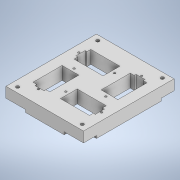
# Autodesk Inventor part: Fuehrungsgrundplatte_V2
Saved by Autodesk Inventor 2022 (Build 260153000, 153)
## iProperties
Created: 2022-04-21
Part Number: Fuehrungsgrundplatte_V2
Material: Generisch
Document SubType Name: Modeling
Designer: 123St
Density: 1 g/cm^3
Appearance: Vorgabe
Author: 123St
Autodesk Inventor part; units mm, degrees
ref_plane "YZ Plane" through (0, 0, 0) normal (1, 0, 0) x (0, 1, 0)
ref_plane "XZ Plane" through (0, 0, 0) normal (0, 1, 0) x (-1, 0, 0)
ref_plane "XY Plane" through (0, 0, 0) normal (0, 0, 1) x (1, 0, 0)
sketch "Skizze1" plane through (0, 0, 0) normal (0, 1, 0) x (-1, 0, 0)
  line L0 (30, -35) -> (-30, -35)
  line L1 (-30, -35) -> (-30, 35)
  line L2 (-30, 35) -> (30, 35)
  line L3 (30, 35) -> (30, -35)
  line L4 (30, -35) -> (-30, 35) construction
  line L5 (-30, -35) -> (30, 35) construction
  point P0 (0, 0)
  dimension "d0" = 60
  dimension "d1" = 70
  constraints: 12 end point, 2 midpoint, 2 parallel, 1 horizontal, 1 perpendicular
  measures "d0" distance of L1.end L2.end
  measures "d1" distance of L0.end L1.end
extrude "Extrusion1" add sketch "Skizze1" along normal blind 10
sketch "Skizze2" plane through (0, 10, 0) normal (0, 1, 0) x (1, 0, 0)
  circle A0 centre (-15.75, 15.75) radius 1.75
  circle A1 centre (15.75, 15.75) radius 1.75
  circle A2 centre (15.75, -15.75) radius 1.75
  circle A3 centre (-15.75, -15.75) radius 1.75
  line L0 (42, 0) -> (-42, 0) projected
  line L1 (0, 49) -> (0, -49) projected
  point P0 (0, 0)
  dimension "d4" = 31.5
  dimension "d5" = 31.5
  dimension "d6" = 15.75
  dimension "d7" = 31.5
  dimension "d8" = 31.5
  dimension "d9" = 15.75
  dimension "d10" = 15.75
  dimension "d11" = 15.75
  dimension "d12" = 3.5
  dimension "d13" = 3.5
  dimension "d14" = 3.5
  dimension "d15" = 3.5
  constraints: 4 centre point
  measures "d4" distance of A0.centre A1.centre
  measures "d5" distance of A2.centre A1.centre
  measures "d6" distance from line of L0 A2.centre
  measures "d7" distance of A3.centre A2.centre
  measures "d8" distance of A0.centre A3.centre
  measures "d9" distance from line of A2.centre L1
  measures "d10" distance from line of L0 A0.centre
  measures "d11" distance from line of L0 A1.centre
  measures "d12" diameter of A0
  measures "d13" diameter of A1
  measures "d14" diameter of A2
  measures "d15" diameter of A3
extrude "Extrusion2" cut sketch "Skizze2" against normal blind 10
sketch "Skizze3" plane through (0, 10, 0) normal (0, 1, 0) x (1, 0, 0)
  circle A0 centre (-15.75, 15.75) radius 1.75 projected
  circle A1 centre (-15.75, 15.75) radius 5
  circle A2 centre (15.75, 15.75) radius 1.75 projected
  circle A3 centre (15.75, 15.75) radius 5
  circle A4 centre (15.75, -15.75) radius 1.75 projected
  circle A5 centre (15.75, -15.75) radius 5
  circle A6 centre (-15.75, -15.75) radius 1.75 projected
  circle A7 centre (-15.75, -15.75) radius 5
  point P0 (0, 0)
  dimension "d18" = 10
  dimension "d19" = 10
  dimension "d20" = 10
  dimension "d21" = 10
  constraints: 4 centre point, 4 coincident
  measures "d18" diameter of A1
  measures "d19" diameter of A3
  measures "d20" diameter of A7
  measures "d21" diameter of A5
extrude "Extrusion3" cut sketch "Skizze3" against normal blind 7 contours A0 | A1 | A2 | A3 | A4 | A5 | A6 | A7
sketch "Skizze6" plane through (0, 0, 0) normal (0, 1, 0) x (-1, 0, 0)
  line L0 (37.5, 25) -> (-37.5, 25)
  line L1 (37.5, -25) -> (-37.5, -25)
  line L2 (37.5, 40) -> (15, 40)
  line L3 (15, 40) -> (15, 30)
  line L4 (-37.5, 40) -> (-15, 40)
  line L5 (-15, 40) -> (-15, 30)
  line L6 (0, -45.47) -> (0, 45.495) projected
  line L7 (37.5, -40) -> (15, -40)
  line L8 (15, -40) -> (15, -30)
  line L9 (-37.5, -40) -> (-15, -40)
  line L10 (-15, -40) -> (-15, -30)
  line L11 (-15, 30) -> (15, 30)
  line L12 (-15, -30) -> (15, -30)
  line L13 (-37.5, 25) -> (-37.5, 40)
  line L14 (37.5, 40) -> (37.5, 25)
  line L15 (-37.5, -25) -> (-37.5, -40)
  line L16 (-30, 35) -> (-30, -35) projected
  line L17 (37.5, -25) -> (37.5, -40)
  point P0 (0, 0)
  dimension "d37" = 10
  dimension "d38" = 15
  dimension "d39" = 15
  dimension "d40" = 75
  dimension "d43" = 10
  dimension "d44" = 15
  dimension "d45" = 15
  dimension "d46" = 22.5
  dimension "d47" = 22.5
  dimension "d48" = 22.5
  dimension "d49" = 75
  dimension "d50" = 22.5
  dimension "d76" = 5
  dimension "d77" = 25
  dimension "d78" = 5
  dimension "d79" = 25
  constraints: 32 end point, 4 parallel, 2 horizontal, 2 point on line, 2 vertical
  measures "d37" distance of L4.end L5.end
  measures "d38" distance between parallel lines of L6 L3
  measures "d39" distance between parallel lines of L6 L5
  measures "d40" distance of L0.start L0.end
  measures "d43" distance of L9.end L10.end
  measures "d44" distance between parallel lines of L10 L6
  measures "d45" distance between parallel lines of L6 L8
  measures "d46" distance of L4.start L4.end
  measures "d47" distance of L2.start L2.end
  measures "d48" distance of L7.start L7.end
  measures "d49" distance of L1.start L1.end
  measures "d50" distance of L9.start L9.end
  measures "d76" distance between parallel lines of L0 L11
  measures "d77" distance from line of L0 point (0, 0)
  measures "d78" distance between parallel lines of L12 L1
  measures "d79" distance from line of point (0, 0) L1
extrude "Extrusion6" cut sketch "Skizze6" along normal blind 2 contours L0 L6 L11 L3 L2 L14 | L0 L13 L4 L5 L11 L6 | L6 L12 L10 L9 L15 L1 | L1 L17 L7 L8 L12 L6
sketch "Skizze7" plane through (0, 2, 0) normal (0, -1, 0) x (1, 0, 0)
  circle A0 centre (-22.5, 30) radius 1.25
  circle A1 centre (22.5, 30) radius 1.25
  circle A2 centre (22.5, -30) radius 1.25
  circle A3 centre (-22.5, -30) radius 1.25
  line L0 (0, 49) -> (0, -49) projected
  line L1 (-42, 0) -> (42, 0) projected
  point P0 (0, 0)
  dimension "d55" = 45
  dimension "d56" = 22.5
  dimension "d57" = 60
  dimension "d58" = 45
  dimension "d59" = 60
  dimension "d60" = 30
  dimension "d61" = 30
  dimension "d62" = 2.5
  dimension "d63" = 2.5
  dimension "d64" = 2.5
  dimension "d65" = 2.5
  dimension "d71" = 22.5
  constraints: 4 centre point
  measures "d55" distance of A1.centre A0.centre
  measures "d56" distance from line of L0 A0.centre
  measures "d57" distance of A3.centre A0.centre
  measures "d58" distance of A2.centre A3.centre
  measures "d59" distance of A1.centre A2.centre
  measures "d60" distance from line of L1 A0.centre
  measures "d61" distance from line of L1 A1.centre
  measures "d62" diameter of A0
  measures "d63" diameter of A1
  measures "d64" diameter of A2
  measures "d65" diameter of A3
  measures "d71" distance from line of L0 A3.centre
extrude "Extrusion7" cut sketch "Skizze7" against normal blind 6
sketch "Skizze9" plane through (0, 10, 0) normal (0, 1, 0) x (1, 0, 0)
  line L0 (-9.25, -21.85) -> (-22.25, -21.85)
  line L1 (-22.25, -21.85) -> (-22.25, 0.65)
  line L2 (-22.25, 0.65) -> (-9.25, 0.65)
  line L3 (-9.25, 0.65) -> (-9.25, -21.85)
  circle A0 centre (-15.75, -15.75) radius 1.75 projected
  line L4 (21.85, -22.25) -> (-0.65, -22.25)
  line L5 (-0.65, -22.25) -> (-0.65, -9.25)
  line L6 (-0.65, -9.25) -> (21.85, -9.25)
  line L7 (21.85, -9.25) -> (21.85, -22.25)
  line L8 (22.25, 21.85) -> (9.25, 21.85)
  line L9 (9.25, 21.85) -> (9.25, -0.65)
  line L10 (9.25, -0.65) -> (22.25, -0.65)
  line L11 (22.25, -0.65) -> (22.25, 21.85)
  circle A1 centre (15.75, 15.75) radius 1.75 projected
  line L12 (-21.85, 9.5) -> (0.65, 9.5)
  line L13 (0.65, 9.5) -> (0.65, 22.5)
  line L14 (0.65, 22.5) -> (-21.85, 22.5)
  line L15 (-21.85, 22.5) -> (-21.85, 9.5)
  circle A2 centre (15.75, -15.75) radius 1.75 projected
  point P0 (0, 0)
  point P1 (-15.75, 16)
  dimension "d80" = 13
  dimension "d81" = 22.5
  dimension "d82" = 6.5
  dimension "d83" = 6.1
  dimension "d97" = 13
  dimension "d99" = 22.5
  dimension "d101" = 13
  dimension "d102" = 6.5
  dimension "d103" = 6.1
  dimension "d104" = 22.5
  dimension "d105" = 13
  dimension "d106" = 22.5
  dimension "d107" = 6.1
  dimension "d108" = 6.5
  dimension "d164" = 6.5
  constraints: 32 end point, 8 parallel, 4 horizontal, 4 perpendicular
  measures "d80" distance of L0.start L0.end
  measures "d81" distance of L0.end L1.end
  measures "d82" distance from line of A0.centre L1
  measures "d83" distance from line of A0.centre L0
  measures "d97" distance of L6.end L4.start
  measures "d99" distance of L4.start L4.end
  measures "d101" distance of L8.start L8.end
  measures "d102" distance from line of L9 A1.centre
  measures "d103" distance from line of L8 A1.centre
  measures "d104" distance of L8.end L9.end
  measures "d105" distance between parallel lines of L14 L12
  measures "d106" distance of L13.end L14.end
  measures "d107" distance from line of L15 point (-15.75, 16)
  measures "d108" distance from line of L12 point (-15.75, 16)
  measures "d164" distance from line of L6 A2.centre
extrude "Extrusion9" cut sketch "Skizze9" against normal blind 10 contours L0 L1 L2 L3 | L4 L5 L6 L7 | L11 L10 L9 L8 | A1 | L15 L14 L13 L12 | A2
sketch "Skizze10" plane through (0, 10, 0) normal (0, 1, 0) x (1, 0, 0)
  circle A0 centre (-3.25, -15.5) radius 0.75
  circle A1 centre (24.45, -15.5) radius 0.75
  circle A2 centre (15.5, -3.25) radius 0.75
  circle A3 centre (15.5, 24.45) radius 0.75
  circle A4 centre (3.25, 15.75) radius 0.75
  circle A5 centre (-24.45, 15.75) radius 0.75
  circle A6 centre (-15.5, 3.25) radius 0.75
  circle A7 centre (-15.5, -24.45) radius 0.75
  line L0 (-22.25, 0.65) -> (-9.25, 0.65) projected
  line L1 (-9.25, -21.85) -> (-22.25, -21.85) projected
  line L2 (-21.85, 9.5) -> (-21.85, 22.5) projected
  line L3 (0.65, 22.5) -> (0.65, 9.5) projected
  line L4 (9.25, 21.85) -> (22.25, 21.85) projected
  line L5 (22.25, -0.65) -> (9.25, -0.65) projected
  line L6 (21.85, -9.25) -> (21.85, -22.25) projected
  line L7 (-0.65, -22.25) -> (-0.65, -9.25) projected
  line L8 (-9.25, 0.65) -> (-9.25, -21.85) projected
  line L9 (-0.65, -9.25) -> (21.85, -9.25) projected
  line L10 (9.25, -0.65) -> (9.25, 21.85) projected
  line L11 (0.65, 9.5) -> (-21.85, 9.5) projected
  point P0 (0, 0)
  dimension "d109" = 1.5
  dimension "d110" = 1.5
  dimension "d111" = 1.5
  dimension "d112" = 1.5
  dimension "d113" = 1.5
  dimension "d114" = 1.5
  dimension "d115" = 1.5
  dimension "d116" = 1.5
  dimension "d117" = 2.6
  dimension "d118" = 2.6
  dimension "d119" = 2.6
  dimension "d120" = 2.6
  dimension "d121" = 2.6
  dimension "d122" = 2.6
  dimension "d123" = 2.6
  dimension "d124" = 2.6
  dimension "d125" = 6.25
  dimension "d126" = 6.25
  dimension "d127" = 6.25
  dimension "d128" = 6.25
  dimension "d130" = 6.25
  dimension "d131" = 6.25
  dimension "d132" = 6.25
  dimension "d133" = 6.25
  constraints: 8 centre point
  measures "d109" diameter of A7
  measures "d110" diameter of A0
  measures "d111" diameter of A1
  measures "d112" diameter of A2
  measures "d113" diameter of A4
  measures "d114" diameter of A3
  measures "d115" diameter of A5
  measures "d116" diameter of A6
  measures "d117" distance from line of L0 A6.centre
  measures "d118" distance from line of L1 A7.centre
  measures "d119" distance from line of L2 A5.centre
  measures "d120" distance from line of L3 A4.centre
  measures "d121" distance from line of L4 A3.centre
  measures "d122" distance from line of L5 A2.centre
  measures "d123" distance from line of L6 A1.centre
  measures "d124" distance from line of L7 A0.centre
  measures "d125" distance from line of L8 A6.centre
  measures "d126" distance from line of A7.centre L8
  measures "d127" distance from line of L9 A0.centre
  measures "d128" distance from line of A1.centre L9
  measures "d130" distance from line of L10 A3.centre
  measures "d131" distance from line of L11 A4.centre
  measures "d132" distance from line of L11 A5.centre
  measures "d133" distance from line of L10 A2.centre
extrude "Extrusion10" cut sketch "Skizze10" against normal blind 5
sketch "Skizze11" plane through (0, 10, 0) normal (0, 1, 0) x (1, 0, 0)
  circle A0 centre (25, -31) radius 1.25
  circle A1 centre (-25, -31) radius 1.25
  circle A2 centre (-25, 31) radius 1.25
  circle A3 centre (25, 31) radius 1.25
  line L0 (-30, -35) -> (30, -35) projected
  line L1 (30, -35) -> (30, 35) projected
  point P0 (0, 0)
  dimension "d136" = 50
  dimension "d137" = 62
  dimension "d138" = 50
  dimension "d139" = 62
  dimension "d140" = 4
  dimension "d141" = 5
  dimension "d142" = 5
  dimension "d143" = 4
  dimension "d144" = 2.5
  dimension "d145" = 2.5
  dimension "d146" = 2.5
  dimension "d147" = 2.5
  constraints: 4 centre point
  measures "d136" distance of A1.centre A0.centre
  measures "d137" distance of A3.centre A0.centre
  measures "d138" distance of A2.centre A3.centre
  measures "d139" distance of A2.centre A1.centre
  measures "d140" distance from line of L0 A1.centre
  measures "d141" distance from line of L1 A0.centre
  measures "d142" distance from line of L1 A3.centre
  measures "d143" distance from line of L0 A0.centre
  measures "d144" diameter of A0
  measures "d145" diameter of A1
  measures "d146" diameter of A2
  measures "d147" diameter of A3
extrude "Extrusion11" cut sketch "Skizze11" against normal blind 5
sketch "Skizze12" plane through (0, 10, 0) normal (0, 1, 0) x (1, 0, 0)
  line L0 (-21.85, 22.5) -> (-21.85, 9.5) projected
  line L1 (-21.85, 12.5) -> (-23.35, 12.5)
  line L2 (-23.35, 12.5) -> (-23.35, 19.5)
  line L3 (-23.35, 19.5) -> (-21.85, 19.5)
  line L4 (-21.85, 19.5) -> (-21.85, 12.5)
  line L5 (9.25, 21.85) -> (22.25, 21.85) projected
  line L6 (19.25, 21.85) -> (12.25, 21.85)
  line L7 (12.25, 21.85) -> (12.25, 23.35)
  line L8 (12.25, 23.35) -> (19.25, 23.35)
  line L9 (19.25, 23.35) -> (19.25, 21.85)
  line L10 (21.85, -9.25) -> (21.85, -22.25) projected
  line L11 (21.85, -19.25) -> (23.35, -19.25)
  line L12 (23.35, -19.25) -> (23.35, -12.25)
  line L13 (23.35, -12.25) -> (21.85, -12.25)
  line L14 (21.85, -12.25) -> (21.85, -19.25)
  line L15 (-9.25, -21.85) -> (-22.25, -21.85) projected
  line L16 (-12.25, -21.85) -> (-19.25, -21.85)
  line L17 (-19.25, -21.85) -> (-19.25, -23.35)
  line L18 (-19.25, -23.35) -> (-12.25, -23.35)
  line L19 (-12.25, -23.35) -> (-12.25, -21.85)
  line L20 (21.85, -22.25) -> (-0.65, -22.25) projected
  line L21 (-0.65, -9.25) -> (21.85, -9.25) projected
  line L22 (-9.25, 0.65) -> (-9.25, -21.85) projected
  line L23 (-22.25, -21.85) -> (-22.25, 0.65) projected
  line L24 (-21.85, 22.5) -> (0.65, 22.5) projected
  line L25 (0.65, 9.5) -> (-21.85, 9.5) projected
  line L26 (9.25, -0.65) -> (9.25, 21.85) projected
  line L27 (22.25, 21.85) -> (22.25, -0.65) projected
  point P0 (0, 0)
  point P1 (-21.85, 19.5)
  dimension "d150" = 3
  dimension "d151" = 3
  dimension "d152" = 1.5
  dimension "d153" = 3
  dimension "d154" = 3
  dimension "d155" = 1.5
  dimension "d156" = 3
  dimension "d157" = 3
  dimension "d158" = 1.5
  dimension "d159" = 3
  dimension "d160" = 3
  dimension "d161" = 1.5
  constraints: 32 end point, 8 parallel, 4 horizontal, 4 perpendicular, 4 point on line
  measures "d150" distance between parallel lines of L20 L11
  measures "d151" distance between parallel lines of L21 L13
  measures "d152" distance of L12.end L13.end
  measures "d153" distance from line of L22 L16.start
  measures "d154" distance between parallel lines of L23 L17
  measures "d155" distance of L16.end L17.end
  measures "d156" distance between parallel lines of L24 L3
  measures "d157" distance between parallel lines of L25 L1
  measures "d158" distance of L2.end L3.end
  measures "d159" distance between parallel lines of L26 L7
  measures "d160" distance between parallel lines of L27 L9
  measures "d161" distance of L8.end L6.start
extrude "Extrusion12" cut sketch "Skizze12" against normal blind 10
equation "\"d6\" = 0.5 * d5"
equation "\"d9\" = 0.5 * d7"
equation "\"d10\" = 0.5 * d8"
equation "\"d11\" = 0.5 * d5"
equation "\"d56\" = 0.5 * d55"
equation "\"d60\" = 0.5 * d57"
equation "\"d61\" = 0.5 * d59"
equation "\"d71\" = 0.5 * d58"
equation "\"d82\" = 0.5 * d80"
equation "\"d102\" = 0.5 * d101"
equation "\"d108\" = 0.5 * d105"
equation "\"d164\" = 0.5 * d97"
